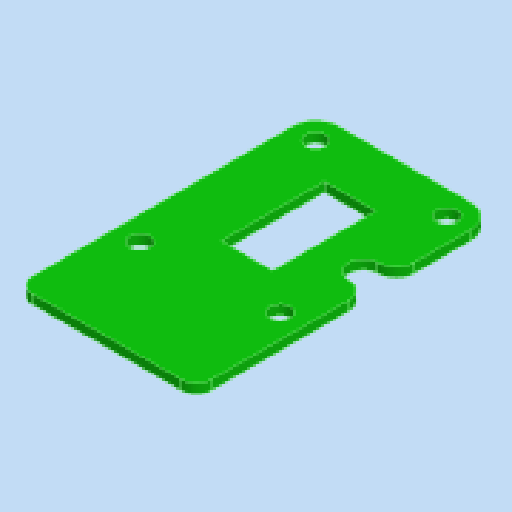
# Autodesk Inventor part: sensor_pcb
Saved by Autodesk Inventor 2024 (Build 280153000, 153)
## iProperties
Created: 2025-05-06
Part Number: sensor_pcb
Material: Generic
Document SubType Name: Modeling
Designer: XxPan
Density: 1 g/cm^3
Appearance: Default
Author: XxPan
Autodesk Inventor part; units mm, degrees
ref_plane "YZ Plane" through (0, 0, 0) normal (1, 0, 0) x (0, 1, 0)
ref_plane "XZ Plane" through (0, 0, 0) normal (0, 1, 0) x (-1, 0, 0)
ref_plane "XY Plane" through (0, 0, 0) normal (0, 0, 1) x (1, 0, 0)
sketch "Sketch1" plane through (0, 0, 0) normal (0, 1, 0) x (-1, 0, 0)
  line L0 (12.5, 25) -> (-12.5, 25)
  line L1 (-11, -25) -> (11, -25)
  line L2 (15, -21) -> (15, 22.5)
  line L3 (22.1598, 0) -> (-22.1598, 0) construction
  line L4 (0, -36.0977) -> (0, 35.787) construction
  arc A0 (-15, -21) -> (-11, -25) centre (-11, -21) ccw
  arc A1 (11, -25) -> (15, -21) centre (11, -21) ccw
  arc A2 (-12.5, 25) -> (-15, 22.5) centre (-12.5, 22.5) ccw
  arc A3 (15, 22.5) -> (12.5, 25) centre (12.5, 22.5) ccw
  line L5 (-15, 22.5) -> (-15, -21)
  point P0 (0, 0)
  point P1 (15, 25)
  point P2 (-15, -25)
  point P3 (-15, 25)
  point P4 (15, -25)
  point P5 (-15, 0)
  dimension "d6" = 15
  dimension "d10" = 4
  dimension "d11" = 2.5
  dimension "d15" = 15
  dimension "d35" = 50
  constraints: 8 end point, 8 point on circle, 8 point on line, 8 tangent, 4 centre point, 2 equal radius, 2 parallel, 1 horizontal, 1 perpendicular, 1 other
  measures "d6" distance between parallel lines of L4 L2
  measures "d10" radius of A0
  measures "d11" radius of A2
  measures "d15" distance between parallel lines of L4 L5
  measures "d35" distance between parallel lines of L1 L0
extrude "Extrusion1" add sketch "Sketch1" along normal blind 1.6
sketch "Sketch2" plane through (0, 1.6, 0) normal (0, 1, 0) x (1, 0, 0)
  line L0 (15, -22.5) -> (15, 21) projected
  line L1 (-15, 21) -> (-15, -22.5) projected
  line L2 (-12.5, -25) -> (12.5, -25) projected
  arc A0 (15, 21) -> (11, 25) centre (11, 21) ccw projected
  arc A1 (-11, 25) -> (-15, 21) centre (-11, 21) ccw projected
  point P0 (0, 0)
  point P1 (-11, -8.5)
  point P2 (11, -7)
  dimension "d36" = 28
  dimension "d37" = 1.5
  constraints: 2 coincident, 2 vertical alignment, 1 horizontal alignment
  measures "d36" distance of point (11, 21) point (11, -7)
  measures "d37" vertical distance of point (11, -7) point (-11, -8.5)
hole "Hole1" at (11, 1.6, -21) at (-11, 1.6, -21) at (-11, 1.6, 8.5) at (11, 1.6, 7) direction (0, -1, 0) diameter 3.4 end through all
sketch "Sketch3" plane through (0, 1.6, 0) normal (0, 1, 0) x (1, 0, 0)
  line L0 (4.3, -1.51) -> (-4.3, -1.51)
  line L1 (-4.3, -1.51) -> (-4.3, 15.75)
  line L2 (-4.3, 15.75) -> (4.3, 15.75)
  line L3 (4.3, 15.75) -> (4.3, -1.51)
  line L4 (0, 35) -> (0, -35) construction
  line L5 (11, 25) -> (-11, 25) projected
  point P0 (0, 0)
  dimension "d29" = 9.25
  dimension "d30" = 8.6
  dimension "d31" = 17.26
  constraints: 8 end point, 2 parallel, 1 horizontal, 1 perpendicular, 1 other
  measures "d29" distance between parallel lines of L5 L2
  measures "d30" distance of L1.end L2.end
  measures "d31" distance of L0.end L1.end
extrude "Extrusion2" cut sketch "Sketch3" against normal through all
sketch "Sketch5" plane through (0, 1.6, 0) normal (0, 1, 0) x (1, 0, 0)
  line L0 (15, -22.5) -> (15, 21) projected
  arc A0 (12, 8.5) -> (12, 3.5) centre (12, 6) ccw
  line L1 (11, 25) -> (-11, 25) projected
  arc A1 (15, 0.5) -> (12, 3.5) centre (12, 0.5) ccw
  arc A2 (12, 8.5) -> (15, 11.5) centre (12, 11.5) ccw
  point P0 (0, 0)
  dimension "d47" = 5
  dimension "d48" = 3
  dimension "d49" = 19
  constraints: 6 point on circle, 4 tangent, 3 centre point, 2 point on line, 2 vertical alignment
  measures "d47" diameter of A0
  measures "d48" distance from line of L0 A0.centre
  measures "d49" distance from line of L1 A0.centre
extrude "Extrusion3" cut sketch "Sketch5" against normal through all
body "Solid1"
